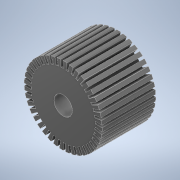
# Autodesk Inventor part: gear(1 inch)
Saved by Autodesk Inventor 2022 (Build 260153070, 153G)
## iProperties
Created: 2021-07-02
Part Number: gear(1 inch)
Material: Acetal Resin, Black
Document SubType Name: Modeling
Designer: hp
Density: 1.425 g/cm^3
Appearance: Smooth - Black
Author: hp
Autodesk Inventor part; units mm, degrees
ref_plane "YZ Plane" through (0, 0, 0) normal (1, 0, 0) x (0, 1, 0)
ref_plane "XZ Plane" through (0, 0, 0) normal (0, 1, 0) x (-1, 0, 0)
ref_plane "XY Plane" through (0, 0, 0) normal (0, 0, 1) x (1, 0, 0)
sketch "Sketch1" plane through (0, 0, 0) normal (0, 0, 1) x (1, 0, 0)
  circle A0 centre (0, 0) radius 12.7
  dimension "d0" = 25.4
  constraints: 1 centre point, 1 coincident
  measures "d0" diameter of A0
extrude "Extrusion1" add sketch "Sketch1" along normal blind 17.5
sketch "Sketch2" plane through (0, 0, 17.5) normal (0, 0, 1) x (1, 0, 0)
  circle A0 centre (0, 0) radius 12.7
  line L0 (-12.7, 0) -> (-10.4428, 0)
  line L1 (-10.4428, 0) -> (-10.4428, -0.7447)
  line L2 (-10.4428, -0.7447) -> (-12.7, -0.7447)
  line L3 (-12.7, -0.7447) -> (-12.7, 0)
  line L4 (-12.5436, -1.9867) -> (-10.3142, -1.6336)
  line L5 (-10.3142, -1.6336) -> (-10.1977, -2.3692)
  line L6 (-10.1977, -2.3692) -> (-12.4271, -2.7223)
  line L7 (-12.4271, -2.7223) -> (-12.5436, -1.9867)
  line L8 (-12.0784, -3.9245) -> (-9.9317, -3.227)
  line L9 (-9.9317, -3.227) -> (-9.7015, -3.9353)
  line L10 (-9.7015, -3.9353) -> (-11.8483, -4.6328)
  line L11 (-11.8483, -4.6328) -> (-12.0784, -3.9245)
  line L12 (-11.3158, -5.7657) -> (-9.3046, -4.7409)
  line L13 (-9.3046, -4.7409) -> (-8.9665, -5.4045)
  line L14 (-8.9665, -5.4045) -> (-10.9777, -6.4292)
  line L15 (-10.9777, -6.4292) -> (-11.3158, -5.7657)
  line L16 (-10.2745, -7.4649) -> (-8.4484, -6.1381)
  line L17 (-8.4484, -6.1381) -> (-8.0106, -6.7406)
  line L18 (-8.0106, -6.7406) -> (-9.8368, -8.0674)
  line L19 (-9.8368, -8.0674) -> (-10.2745, -7.4649)
  line L20 (-8.9803, -8.9803) -> (-7.3841, -7.3841)
  line L21 (-7.3841, -7.3841) -> (-6.8575, -7.9108)
  line L22 (-6.8575, -7.9108) -> (-8.4536, -9.5069)
  line L23 (-8.4536, -9.5069) -> (-8.9803, -8.9803)
  line L24 (-7.4649, -10.2745) -> (-6.1381, -8.4484)
  line L25 (-6.1381, -8.4484) -> (-5.5356, -8.8861)
  line L26 (-5.5356, -8.8861) -> (-6.8624, -10.7123)
  line L27 (-6.8624, -10.7123) -> (-7.4649, -10.2745)
  line L28 (-5.7657, -11.3158) -> (-4.7409, -9.3046)
  line L29 (-4.7409, -9.3046) -> (-4.0773, -9.6427)
  line L30 (-4.0773, -9.6427) -> (-5.1021, -11.6539)
  line L31 (-5.1021, -11.6539) -> (-5.7657, -11.3158)
  line L32 (-3.9245, -12.0784) -> (-3.227, -9.9317)
  line L33 (-3.227, -9.9317) -> (-2.5187, -10.1618)
  line L34 (-2.5187, -10.1618) -> (-3.2162, -12.3086)
  line L35 (-3.2162, -12.3086) -> (-3.9245, -12.0784)
  line L36 (-1.9867, -12.5436) -> (-1.6336, -10.3142)
  line L37 (-1.6336, -10.3142) -> (-0.898, -10.4307)
  line L38 (-0.898, -10.4307) -> (-1.2511, -12.6601)
  line L39 (-1.2511, -12.6601) -> (-1.9867, -12.5436)
  line L40 (0, -12.7) -> (0, -10.4428)
  line L41 (0, -10.4428) -> (0.7447, -10.4428)
  line L42 (0.7447, -10.4428) -> (0.7447, -12.7)
  line L43 (0.7447, -12.7) -> (0, -12.7)
  line L44 (1.9867, -12.5436) -> (1.6336, -10.3142)
  line L45 (1.6336, -10.3142) -> (2.3692, -10.1977)
  line L46 (2.3692, -10.1977) -> (2.7223, -12.4271)
  line L47 (2.7223, -12.4271) -> (1.9867, -12.5436)
  line L48 (3.9245, -12.0784) -> (3.227, -9.9317)
  line L49 (3.227, -9.9317) -> (3.9353, -9.7015)
  line L50 (3.9353, -9.7015) -> (4.6328, -11.8483)
  line L51 (4.6328, -11.8483) -> (3.9245, -12.0784)
  line L52 (5.7657, -11.3158) -> (4.7409, -9.3046)
  line L53 (4.7409, -9.3046) -> (5.4045, -8.9665)
  line L54 (5.4045, -8.9665) -> (6.4292, -10.9777)
  line L55 (6.4292, -10.9777) -> (5.7657, -11.3158)
  line L56 (7.4649, -10.2745) -> (6.1381, -8.4484)
  line L57 (6.1381, -8.4484) -> (6.7406, -8.0106)
  line L58 (6.7406, -8.0106) -> (8.0674, -9.8368)
  line L59 (8.0674, -9.8368) -> (7.4649, -10.2745)
  line L60 (8.9803, -8.9803) -> (7.3841, -7.3841)
  line L61 (7.3841, -7.3841) -> (7.9108, -6.8575)
  line L62 (7.9108, -6.8575) -> (9.5069, -8.4536)
  line L63 (9.5069, -8.4536) -> (8.9803, -8.9803)
  line L64 (10.2745, -7.4649) -> (8.4484, -6.1381)
  line L65 (8.4484, -6.1381) -> (8.8861, -5.5356)
  line L66 (8.8861, -5.5356) -> (10.7123, -6.8624)
  line L67 (10.7123, -6.8624) -> (10.2745, -7.4649)
  line L68 (11.3158, -5.7657) -> (9.3046, -4.7409)
  line L69 (9.3046, -4.7409) -> (9.6427, -4.0773)
  line L70 (9.6427, -4.0773) -> (11.6539, -5.1021)
  line L71 (11.6539, -5.1021) -> (11.3158, -5.7657)
  line L72 (12.0784, -3.9245) -> (9.9317, -3.227)
  line L73 (9.9317, -3.227) -> (10.1618, -2.5187)
  line L74 (10.1618, -2.5187) -> (12.3086, -3.2162)
  line L75 (12.3086, -3.2162) -> (12.0784, -3.9245)
  line L76 (12.5436, -1.9867) -> (10.3142, -1.6336)
  line L77 (10.3142, -1.6336) -> (10.4307, -0.898)
  line L78 (10.4307, -0.898) -> (12.6601, -1.2511)
  line L79 (12.6601, -1.2511) -> (12.5436, -1.9867)
  line L80 (12.7, 0) -> (10.4428, 0)
  line L81 (10.4428, 0) -> (10.4428, 0.7447)
  line L82 (10.4428, 0.7447) -> (12.7, 0.7447)
  line L83 (12.7, 0.7447) -> (12.7, 0)
  line L84 (12.5436, 1.9867) -> (10.3142, 1.6336)
  line L85 (10.3142, 1.6336) -> (10.1977, 2.3692)
  line L86 (10.1977, 2.3692) -> (12.4271, 2.7223)
  line L87 (12.4271, 2.7223) -> (12.5436, 1.9867)
  line L88 (12.0784, 3.9245) -> (9.9317, 3.227)
  line L89 (9.9317, 3.227) -> (9.7015, 3.9353)
  line L90 (9.7015, 3.9353) -> (11.8483, 4.6328)
  line L91 (11.8483, 4.6328) -> (12.0784, 3.9245)
  line L92 (11.3158, 5.7657) -> (9.3046, 4.7409)
  line L93 (9.3046, 4.7409) -> (8.9665, 5.4045)
  line L94 (8.9665, 5.4045) -> (10.9777, 6.4292)
  line L95 (10.9777, 6.4292) -> (11.3158, 5.7657)
  line L96 (10.2745, 7.4649) -> (8.4484, 6.1381)
  line L97 (8.4484, 6.1381) -> (8.0106, 6.7406)
  line L98 (8.0106, 6.7406) -> (9.8368, 8.0674)
  line L99 (9.8368, 8.0674) -> (10.2745, 7.4649)
  line L100 (8.9803, 8.9803) -> (7.3841, 7.3841)
  line L101 (7.3841, 7.3841) -> (6.8575, 7.9108)
  line L102 (6.8575, 7.9108) -> (8.4536, 9.5069)
  line L103 (8.4536, 9.5069) -> (8.9803, 8.9803)
  line L104 (7.4649, 10.2745) -> (6.1381, 8.4484)
  line L105 (6.1381, 8.4484) -> (5.5356, 8.8861)
  line L106 (5.5356, 8.8861) -> (6.8624, 10.7123)
  line L107 (6.8624, 10.7123) -> (7.4649, 10.2745)
  line L108 (5.7657, 11.3158) -> (4.7409, 9.3046)
  line L109 (4.7409, 9.3046) -> (4.0773, 9.6427)
  line L110 (4.0773, 9.6427) -> (5.1021, 11.6539)
  line L111 (5.1021, 11.6539) -> (5.7657, 11.3158)
  line L112 (3.9245, 12.0784) -> (3.227, 9.9317)
  line L113 (3.227, 9.9317) -> (2.5187, 10.1618)
  line L114 (2.5187, 10.1618) -> (3.2162, 12.3086)
  line L115 (3.2162, 12.3086) -> (3.9245, 12.0784)
  line L116 (1.9867, 12.5436) -> (1.6336, 10.3142)
  line L117 (1.6336, 10.3142) -> (0.898, 10.4307)
  line L118 (0.898, 10.4307) -> (1.2511, 12.6601)
  line L119 (1.2511, 12.6601) -> (1.9867, 12.5436)
  line L120 (0, 12.7) -> (0, 10.4428)
  line L121 (0, 10.4428) -> (-0.7447, 10.4428)
  line L122 (-0.7447, 10.4428) -> (-0.7447, 12.7)
  line L123 (-0.7447, 12.7) -> (0, 12.7)
  line L124 (-1.9867, 12.5436) -> (-1.6336, 10.3142)
  line L125 (-1.6336, 10.3142) -> (-2.3692, 10.1977)
  line L126 (-2.3692, 10.1977) -> (-2.7223, 12.4271)
  line L127 (-2.7223, 12.4271) -> (-1.9867, 12.5436)
  line L128 (-3.9245, 12.0784) -> (-3.227, 9.9317)
  line L129 (-3.227, 9.9317) -> (-3.9353, 9.7015)
  line L130 (-3.9353, 9.7015) -> (-4.6328, 11.8483)
  line L131 (-4.6328, 11.8483) -> (-3.9245, 12.0784)
  line L132 (-5.7657, 11.3158) -> (-4.7409, 9.3046)
  line L133 (-4.7409, 9.3046) -> (-5.4045, 8.9665)
  line L134 (-5.4045, 8.9665) -> (-6.4292, 10.9777)
  line L135 (-6.4292, 10.9777) -> (-5.7657, 11.3158)
  line L136 (-7.4649, 10.2745) -> (-6.1381, 8.4484)
  line L137 (-6.1381, 8.4484) -> (-6.7406, 8.0106)
  line L138 (-6.7406, 8.0106) -> (-8.0674, 9.8368)
  line L139 (-8.0674, 9.8368) -> (-7.4649, 10.2745)
  line L140 (-8.9803, 8.9803) -> (-7.3841, 7.3841)
  line L141 (-7.3841, 7.3841) -> (-7.9108, 6.8575)
  line L142 (-7.9108, 6.8575) -> (-9.5069, 8.4536)
  line L143 (-9.5069, 8.4536) -> (-8.9803, 8.9803)
  line L144 (-10.2745, 7.4649) -> (-8.4484, 6.1381)
  line L145 (-8.4484, 6.1381) -> (-8.8861, 5.5356)
  line L146 (-8.8861, 5.5356) -> (-10.7123, 6.8624)
  line L147 (-10.7123, 6.8624) -> (-10.2745, 7.4649)
  line L148 (-11.3158, 5.7657) -> (-9.3046, 4.7409)
  line L149 (-9.3046, 4.7409) -> (-9.6427, 4.0773)
  line L150 (-9.6427, 4.0773) -> (-11.6539, 5.1021)
  line L151 (-11.6539, 5.1021) -> (-11.3158, 5.7657)
  line L152 (-12.0784, 3.9245) -> (-9.9317, 3.227)
  line L153 (-9.9317, 3.227) -> (-10.1618, 2.5187)
  line L154 (-10.1618, 2.5187) -> (-12.3086, 3.2162)
  line L155 (-12.3086, 3.2162) -> (-12.0784, 3.9245)
  line L156 (-12.5436, 1.9867) -> (-10.3142, 1.6336)
  line L157 (-10.3142, 1.6336) -> (-10.4307, 0.898)
  line L158 (-10.4307, 0.898) -> (-12.6601, 1.2511)
  line L159 (-12.6601, 1.2511) -> (-12.5436, 1.9867)
  dimension "d5" = 360
  constraints: 320 end point, 1 horizontal alignment, 323 other
extrude "Extrusion2" cut sketch "Sketch2" against normal through all contours L80 L81 L82 A0 | A0 L82 L83 | L78 L79 A0 | A0 L76 L77 L78 | L84 L85 L86 A0 | A0 L86 L87 | L74 L75 A0 | A0 L72 L73 L74 | L88 L89 L90 A0 | A0 L90 L91 | L70 L71 A0 | A0 L68 L69 L70 | L92 L93 L94 A0 | A0 L94 L95 | L66 L67 A0 | A0 L64 L65 L66 | L96 L97 L98 A0 | A0 L98 L99 | L62 L63 A0 | A0 L60 L61 L62 | L100 L101 L102 A0 | A0 L102 L103 | L58 L59 A0 | A0 L56 L57 L58 | L104 L105 L106 A0 | A0 L106 L107 | L54 L55 A0 | A0 L52 L53 L54 | L108 L109 L110 A0 | A0 L110 L111 | L50 L51 A0 | A0 L48 L49 L50 | L112 L113 L114 A0 | A0 L114 L115 | L46 L47 A0 | A0 L44 L45 L46 | L116 L117 L118 A0 | A0 L118 L119 | L42 L43 A0 | A0 L40 L41 L42 | L120 L121 L122 A0 | A0 L122 L123 | L38 L39 A0 | A0 L36 L37 L38 | L124 L125 L126 A0 | A0 L126 L127 | L34 L35 A0 | A0 L32 L33 L34 | L128 L129 L130 A0 | A0 L130 L131 | L30 L31 A0 | A0 L28 L29 L30 | L132 L133 L134 A0 | A0 L134 L135 | L26 L27 A0 | A0 L24 L25 L26 | L136 L137 L138 A0 | A0 L138 L139 | L22 L23 A0 | A0 L20 L21 L22 | L140 L141 L142 A0 | A0 L142 L143 | L18 L19 A0 | A0 L16 L17 L18 | L144 L145 L146 A0 | A0 L146 L147 | L14 L15 A0 | A0 L12 L13 L14 | L148 L149 L150 A0 | A0 L150 L151 | L10 L11 A0 | A0 L8 L9 L10 | L152 L153 L154 A0 | A0 L154 L155 | L6 L7 A0 | A0 L4 L5 L6 | L156 L157 L158 A0 | A0 L158 L159 | L2 L3 A0 | A0 L0 L1 L2
sketch "Sketch3" plane through (0, 0, 17.5) normal (0, 0, 1) x (1, 0, 0)
  point P0 (0, 0)
  point P1 (0, 0)
  constraints: 1 coincident
hole "Hole1" at (0, 0, 17.5) direction (0, 0, -1) diameter 6 end through all
sketch "Sketch4" plane through (0, 0, 0) normal (0, 1, 0) x (-1, 0, 0)
  point P0 (0, 0)
body "Solid1"
